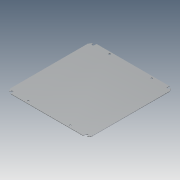
# Autodesk Inventor part: AE 1050_01_00 MontagePlatte
Saved by Autodesk Inventor 2016 (Build 200138000, 138)
## iProperties
Category: PARTsolutions
Company: RITTAL
Created: 2014-04-04
Part Number: AE 1050_01_00 MontagePlatte
Catalog Web Link: www.cadenas.de
Description: Montageplatte AE-Montageplatte AE
Vendor: RITTAL
Document SubType Name: Modeling
Designer: PARTuser1
Manufacturer: RITTAL
Density: 1 g/cm^3
Material: Generic
Appearance: RGB(195.00000357627781,201.00000321865156,196.00000351667384)
PSOL_IDENT_0: {$CADENAS_DATA\23d-libs\rittal\schaltschranksys\kompakt_schaltschr\ae\parts_ae\montageplatte_ae.prj}
PSOL_IDENT_1: ,187 {VTYP=3D},{NB=1050_02_08 (1)},{LINA=1050_02_08 (1)},{NN=Montageplatte AE},{DATE=16.04.2012 12:4
PSOL_IDENT_2: 1:10},{GEOMDATE=31.01.2012 08:39:00},{VERSION=},{LINEID=450},{LINESUBID=-1},{WBVAR=DETAIL}  {NB=1050
PSOL_IDENT_3: _02_08 (1)},{LINA=1050_02_08 (1)},{KT=DUMMY},{BEST=1050_02_08},{VERS=2},{DETAIL=1},{Q=449.000},{K=47
PSOL_IDENT_4: 0.000},{A=500.000},{B=500.000},{C=210.000},{D=303.000},{E=113.000},{F=38.000},{G=30.000},{H=445.000}
PSOL_IDENT_5: ,{I=355.000},{P=410.000},{R=495.000},{S=495.000},{T=356.300},{U=425.000},{V=17.000},{W=438.000},{X=4
PSOL_IDENT_6: 11.000},{Y=423.000},{B1=500},{H1=500},{T1=210},{F1=449},{G1=470},{S1=2.5},{GEW=16.8}
CNS_NN: Montageplatte AE
CNS_NT: Montageplatte AE
CNS_NB: 1050_02_08 (1)
CNS_NBSYN: $BEST. ($DETAIL.)
CNS_LINA: 1050_02_08 (1)
CNS_BEST: 1050_02_08
CNS_VERS: 2
CNS_DETAIL: 1
CNS_Q: 449.000
CNS_K: 470.000
CNS_A: 500.000
CNS_B: 500.000
CNS_C: 210.000
CNS_D: 303.000
CNS_E: 113.000
CNS_F: 38.000
CNS_G: 30.000
CNS_H: 445.000
CNS_I: 355.000
CNS_P: 410.000
CNS_R: 495.000
CNS_S: 495.000
CNS_T: 356.300
CNS_U: 425.000
CNS_V: 17.000
CNS_W: 438.000
CNS_X: 411.000
CNS_Y: 423.000
CNS_B1: 500
CNS_H1: 500
CNS_T1: 210
CNS_F1: 449
CNS_G1: 470
CNS_S1: 2.5
CNS_GEW: 16.8
SUPPLIER: RITTAL
ARTICLENO: 1050_02_08 (1)
BOMINFO: 1050_02_08 (1)
CREATOR: CADENAS GmbH
Title: 1050_02_08 (1)
Author: Cadenas PARTsolutions
Comments: Montageplatte AE
Autodesk Inventor part; units mm, degrees
sketch "Skizze_2" plane through (0, 0, 0) normal (0, 0, 1) x (1, 0, 0)
  line L0 (-224.5, 433.5455) -> (-224.5, 11.4545)
  line L1 (-224.5, 11.4545) -> (-215, -5)
  line L2 (-215, -5) -> (-211, -5)
  line L3 (-211, -5) -> (-211, 0)
  arc A0 (-199, 0) -> (-211, 0) centre (-205, 0) ccw
  line L4 (-199, 0) -> (-199, -12.5)
  line L5 (-199, -12.5) -> (199, -12.5)
  line L6 (199, -12.5) -> (199, 0)
  arc A1 (211, 0) -> (199, 0) centre (205, 0) ccw
  line L7 (211, 0) -> (211, -5)
  line L8 (211, -5) -> (215, -5)
  line L9 (215, -5) -> (224.5, 11.4545)
  line L10 (224.5, 11.4545) -> (224.5, 433.5455)
  line L11 (224.5, 433.5455) -> (215, 450)
  line L12 (215, 450) -> (211, 450)
  line L13 (211, 450) -> (211, 445)
  arc A2 (199, 445) -> (211, 445) centre (205, 445) ccw
  line L14 (199, 445) -> (199, 457.5)
  line L15 (199, 457.5) -> (-199, 457.5)
  line L16 (-199, 457.5) -> (-199, 445)
  arc A3 (-211, 445) -> (-199, 445) centre (-205, 445) ccw
  line L17 (-211, 445) -> (-211, 450)
  line L18 (-211, 450) -> (-215, 450)
  line L19 (-215, 450) -> (-224.5, 433.5455)
  circle A4 centre (115, 445) radius 5
  circle A5 centre (115, 0) radius 5
  circle A6 centre (-115, 445) radius 5
  circle A7 centre (-115, 0) radius 5
  constraints: 40 end point, 8 centre point, 8 point on circle
extrude "Extrusion1" add sketch "Skizze_2" against normal blind 2
ref_plane "DPF11_XY" through (224.5, 222.5, 0) normal (0, 0, 1) x (1, 0, 0)
ref_plane "DPF11_YZ" through (224.5, 222.5, 0) normal (1, 0, 0) x (0, 1, 0)
ref_plane "DPF11_ZX" through (224.5, 222.5, 0) normal (0, 1, 0) x (0, 0, 1)
ref_plane "DPF12_XY" through (-224.5, 222.5, 0) normal (0, 0, 1) x (1, 0, 0)
ref_plane "DPF12_YZ" through (-224.5, 222.5, 0) normal (1, 0, 0) x (0, 1, 0)
ref_plane "DPF12_ZX" through (-224.5, 222.5, 0) normal (0, 1, 0) x (0, 0, 1)
ref_plane "DPF21_XY" through (205, 445, 0) normal (0, 0, 1) x (1, 0, 0)
ref_plane "DPF21_YZ" through (205, 445, 0) normal (1, 0, 0) x (0, 1, 0)
ref_plane "DPF21_ZX" through (205, 445, 0) normal (0, 1, 0) x (0, 0, 1)
ref_plane "DPF22_XY" through (-205, 445, 0) normal (0, 0, 1) x (1, 0, 0)
ref_plane "DPF22_YZ" through (-205, 445, 0) normal (1, 0, 0) x (0, 1, 0)
ref_plane "DPF22_ZX" through (-205, 445, 0) normal (0, 1, 0) x (0, 0, 1)
ref_plane "DPG11_XY" through (0, -12.5, 0) normal (0, 0, 1) x (1, 0, 0)
ref_plane "DPG11_YZ" through (0, -12.5, 0) normal (1, 0, 0) x (0, 1, 0)
ref_plane "DPG11_ZX" through (0, -12.5, 0) normal (0, 1, 0) x (0, 0, 1)
ref_plane "DPG12_XY" through (0, 457.5, 0) normal (0, 0, 1) x (1, 0, 0)
ref_plane "DPG12_YZ" through (0, 457.5, 0) normal (1, 0, 0) x (0, 1, 0)
ref_plane "DPG12_ZX" through (0, 457.5, 0) normal (0, 1, 0) x (0, 0, 1)
ref_plane "DPG21_XY" through (205, 0, 0) normal (0, 0, 1) x (1, 0, 0)
ref_plane "DPG21_YZ" through (205, 0, 0) normal (1, 0, 0) x (0, 1, 0)
ref_plane "DPG21_ZX" through (205, 0, 0) normal (0, 1, 0) x (0, 0, 1)
ref_plane "DPG22_XY" through (205, 445, 0) normal (0, 0, 1) x (1, 0, 0)
ref_plane "DPG22_YZ" through (205, 445, 0) normal (1, 0, 0) x (0, 1, 0)
ref_plane "DPG22_ZX" through (205, 445, 0) normal (0, 1, 0) x (0, 0, 1)
ref_plane "montageplatte_XY" through (-205, 0, 0) normal (0, 0, 1) x (1, 0, 0)
ref_plane "montageplatte_YZ" through (-205, 0, 0) normal (1, 0, 0) x (0, 1, 0)
ref_plane "montageplatte_ZX" through (-205, 0, 0) normal (0, 1, 0) x (0, 0, 1)
body "Solid1"
